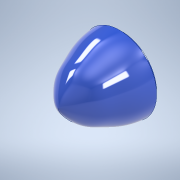
# Autodesk Inventor part: nose
Saved by Autodesk Inventor 2020 (Build 240168000, 168)
## iProperties
Created: 2021-01-23
Part Number: nose
Material: ABS Plastic
Document SubType Name: Modeling
Designer: 0x6f736f646f
Density: 1.06 g/cm^3
Appearance: Smooth - White
Author: 0x6f736f646f
Autodesk Inventor part; units mm, degrees
ref_plane "YZ Plane" through (0, 0, 0) normal (1, 0, 0) x (0, 1, 0)
ref_plane "XZ Plane" through (0, 0, 0) normal (0, 1, 0) x (-1, 0, 0)
ref_plane "XY Plane" through (0, 0, 0) normal (0, 0, 1) x (1, 0, 0)
sketch "Sketch1" plane through (0, 0, 0) normal (1, 0, 0) x (0, 1, 0)
  line L0 (-58, -10) -> (-58.1156, -10)
  line L1 (0, 0) -> (-58, 0)
  line L2 (-50, 0) -> (-50, -4)
  line L3 (-50, -4) -> (-54, -4)
  line L4 (-54, -4) -> (-54, 0)
  line L5 (-54, 0) -> (-58, 0)
  line L6 (-50, 0) -> (-50, 20)
  line L7 (0, 74) -> (0, 96)
  line L8 (-58, 0) -> (-56, 24.2459) construction
  line L9 (-56, 24.2459) -> (-43.6427, 45.1584) construction
  line L10 (-43.6427, 45.1584) -> (-39.7487, 66.7921) construction
  line L11 (-39.7487, 66.7921) -> (-23.0677, 79.9782) construction
  line L12 (-23.0677, 79.9782) -> (-10.7596, 92.3197) construction
  line L13 (-10.7596, 92.3197) -> (0, 96) construction
  spline S0 degree 4 poles (-58, 0) (-56, 24.2459) (-43.6427, 45.1584) (-39.7487, 66.7921) (-23.0677, 79.9782) (-10.7596, 92.3197) (0, 96) knots 1 1 1 1 1 2 3 4 4 4 4 4
  line L14 (-50, 20) -> (-20, 20)
  line L15 (-20, 20) -> (-20, 74)
  line L16 (-20, 74) -> (0, 74)
  line L17 (0, -32.9822) -> (0, 127.8935) projected
  dimension "d25" = 4
  dimension "d26" = 4
  dimension "d27" = 4
  dimension "d29" = 20
  dimension "d31" = 58
  dimension "d32" = 96
  dimension "d33" = 50
  dimension "d34" = 30
  dimension "d35" = 54
  constraints: 22 end point, 4 horizontal, 4 perpendicular, 2 point on line, 1 vertical, 3 other
  measures "d25" distance from line of L1.end L4
  measures "d26" distance of L2.end L3.end
  measures "d27" distance of L3.end L4.end
  measures "d29" distance of L2.start L6.end
  measures "d31" distance of L1.end point (0, 0)
  measures "d32" distance of point (0, 0) L7.end
  measures "d33" distance between parallel lines of L6 L7
  measures "d34" distance of L6.end L14.end
  measures "d35" distance of L14.end L15.end
revolve "Revolution1" add sketch "Sketch1" angle 360 about axis through (0, 0, -10) along (0, 0, 1) contours L2 L3 L4 L1 | L1 S0 L7 L16 L15 L14 L6
body "Solid1"
